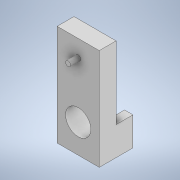
# Autodesk Inventor part: bottom_part
Saved by Autodesk Inventor 2021 (Build 250183000, 183)
## iProperties
Created: 2021-04-02
Part Number: bottom_part
Material: Generic
Document SubType Name: Modeling
Designer: Jawal
Density: 1 g/cm^3
Appearance: Default
Author: Jawal
Autodesk Inventor part; units mm, degrees
ref_plane "YZ Plane" through (0, 0, 0) normal (1, 0, 0) x (0, 1, 0)
ref_plane "XZ Plane" through (0, 0, 0) normal (0, 1, 0) x (-1, 0, 0)
ref_plane "XY Plane" through (0, 0, 0) normal (0, 0, 1) x (1, 0, 0)
sketch "Sketch1" plane through (0, 0, 0) normal (0, 0, 1) x (1, 0, 0)
  line L0 (-12.5, -12.5) -> (12.5, -12.5)
  line L1 (12.5, -12.5) -> (12.5, 47.5)
  line L2 (12.5, 47.5) -> (-12.5, 47.5)
  line L3 (-12.5, 47.5) -> (-12.5, -12.5)
  point P0 (0, 0)
  dimension "d0" = 60
  dimension "d1" = 25
  dimension "d2" = 12.5
  dimension "d5" = 12.5
  constraints: 8 end point, 2 parallel, 1 horizontal, 1 perpendicular
  measures "d0" distance of L0.end L1.end
  measures "d1" distance of L0.start L0.end
  measures "d2" distance from line of L3 point (0, 0)
  measures "d5" distance from line of L0 point (0, 0)
extrude "Extrusion1" add sketch "Sketch1" against normal blind 10
sketch "Sketch2" plane through (0, 0, 0) normal (0, 0, 1) x (1, 0, 0)
  circle A0 centre (0, 37.5) radius 1.5
  point P0 (0, 0)
  dimension "d8" = 3
  dimension "d29" = 37.5
  constraints: 1 centre point
  measures "d8" diameter of A0
  measures "d29" distance of point (0, 0) A0.centre
extrude "Extrusion2" add sketch "Sketch2" along normal blind 6
thread "Thread1" size "M3x0.5" class "6g" standard "ANSI Metric M Profile" full length
sketch "Sketch3" plane through (0, 0, -10) normal (0, 0, -1) x (-1, 0, 0)
  line L0 (-7.5, 4.5) -> (-12.5, 4.5)
  line L1 (-12.5, 47.5) -> (-12.5, -12.5) projected
  line L2 (-12.5, -12.5) -> (12.5, -12.5) projected
  line L3 (-12.5, -12.5) -> (12.5, -12.5)
  line L4 (12.5, -12.5) -> (12.5, 4.5)
  line L5 (12.5, -12.5) -> (12.5, 47.5) projected
  line L6 (7.5, 4.5) -> (12.5, 4.5)
  arc A0 (-7.5, 4.5) -> (7.5, 4.5) centre (0, 4.5) ccw
  point P0 (0, 0)
  dimension "d20" = 17
  dimension "d21" = 5
  dimension "d22" = 5
  dimension "d25" = 7.5
  constraints: 8 end point, 4 point on line, 2 horizontal, 2 point on circle, 1 centre point, 1 perpendicular
  measures "d20" distance of L2.end L4.end
  measures "d21" distance of L6.start L4.end
  measures "d22" distance of L0.start L0.end
  measures "d25" radius of A0
extrude "Extrusion3" add sketch "Sketch3" along normal blind 10
sketch "Sketch5" plane through (0, 0, 0) normal (0, 0, 1) x (1, 0, 0)
  circle A0 centre (0, 4.5) radius 7.5
  point P0 (0, 0)
  dimension "d26" = 15
  constraints: 1 centre point
  measures "d26" diameter of A0
extrude "Extrusion5" cut sketch "Sketch5" against normal blind 10
equation "\"d2\" = 0.5 * d1"
body "Solid1"
